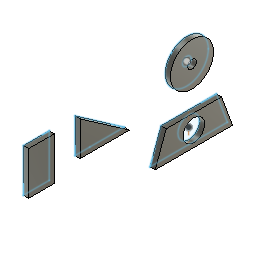
4thLesson v1 (Autodesk Fusion 360 design; units mm, degrees)
Autodesk Fusion 360 part; units mm, degrees
sketch "Sketch1" plane through (0, 0, 0) normal (1, 0, 0) x (0, 1, 0)
  line L0 (10, 10) -> (40, 10)
  line L1 (40, 10) -> (40, 60)
  line L2 (40, 60) -> (10, 60)
  line L3 (10, 60) -> (10, 10)
  line L4 (70, 60) -> (70, 20)
  line L5 (70, 20) -> (87.2389, 20)
  line L6 (87.2389, 20) -> (127.2389, 20)
  line L7 (70, 60) -> (127.2389, 20)
  circle A0 centre (200, 50) radius 25
  circle A1 centre (200, 50) radius 5
  line L8 (170, 0) -> (234.3166, 0)
  line L9 (202.1583, 0) -> (202.1583, -35) construction
  line L10 (202.1583, -35) -> (247.1583, -35)
  line L11 (202.1583, -35) -> (157.1583, -35)
  line L12 (170, 0) -> (157.1583, -35)
  line L13 (234.3166, 0) -> (247.1583, -35)
  circle A2 centre (202.1583, -17.5) radius 12.5
  dimension "d1" = 30
  dimension "d2" = 50
  dimension "d3" = 40
  dimension "d4" = 40
  dimension "d5" = 50
  dimension "d6" = 10
  dimension "d7" = 35
  dimension "d8" = 45
  dimension "d9" = 45
  dimension "d10" = 25
  constraint horizontal L0
  constraint vertical L1
  constraint horizontal L2
  constraint vertical L3
  constraint vertical L4
  constraint perpendicular L4 L5
  constraint perpendicular L4 L6
  constraint concentric A0 A1
  constraint horizontal L8
  constraint midpoint L8 L9.start
  constraint perpendicular L8 L9
  constraint perpendicular L9 L10
  constraint perpendicular L9 L11
  constraint midpoint L9 A2.centre
  measures "d1" distance of L0.start L0.end
  measures "d2" distance of L0.start L2.end
  measures "d3" distance of L4.start L4.end
  measures "d4" distance of L5.end L6.end
  measures "d5" diameter of A0
  measures "d6" diameter of A1
  measures "d7" distance of L9.start L9.end
  measures "d8" distance of L9.end L10.end
  measures "d9" distance of L9.end L11.end
  measures "d10" diameter of A2
extrude "Extrude1" add sketch "Sketch1" along normal blind 6 makes body 1 at (0, 89.0796, 33.3333) makes body 2 at (0, 218.2216, 48.5096) makes body 3 at (0, 20, 43.3333) makes body 4 at (0, 172.2722, -17.5)
